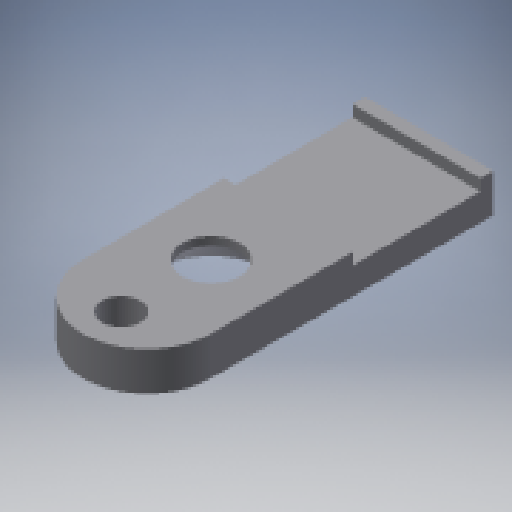
# Autodesk Inventor part: 24_0497_007
Saved by Autodesk Inventor 2024.3 (Build 283343000, 343)
## iProperties
Created: 2024-06-06
Part Number: 24_0497_007
Material: Allgemein
Document SubType Name: Modeling
Designer: Vogel
Density: 1 g/cm^3
Appearance: Vorgabe
Author: Vogel
Autodesk Inventor part; units mm, degrees
ref_plane "YZ Plane" through (0, 0, 0) normal (1, 0, 0) x (0, 1, 0)
ref_plane "XZ Plane" through (0, 0, 0) normal (0, 1, 0) x (-1, 0, 0)
ref_plane "XY Plane" through (0, 0, 0) normal (0, 0, 1) x (1, 0, 0)
sketch "Skizze1" plane through (0, 0, 0) normal (0, 0, 1) x (1, 0, 0)
  line L0 (-7, 0) -> (7, 0) projected
  line L1 (0, -30) -> (0, 5) projected
  line L2 (5, -20) -> (-5, -20)
  line L3 (-5, -20) -> (-5, 0)
  line L4 (-5, 0) -> (5, 0)
  line L5 (5, 0) -> (5, -20)
  line L6 (5, -20) -> (-5, 0) construction
  line L7 (-5, -20) -> (5, 0) construction
  arc A0 (-5, -20) -> (5, -20) centre (0, -20) ccw
  point P0 (0, 0)
  point P1 (0, -10)
  dimension "d0" = 10
  dimension "d1" = 20
  constraints: 12 end point, 2 midpoint, 2 parallel, 2 point on circle, 2 point on line, 2 tangent, 1 centre point, 1 horizontal, 1 perpendicular
  measures "d0" distance between parallel lines of L5 L3
  measures "d1" distance of L2.end L3.end
extrude "Extrusion1" add sketch "Skizze1" along normal blind 3
sketch "Skizze2" plane through (5, -20, 0) normal (1, 0, 0) x (0, 0, -1)
  line L0 (0, 0) -> (0, 20) projected
  line L1 (0, 20) -> (-3, 20) projected
  line L2 (-3, 0) -> (-3, 20) projected
  line L3 (0, 0) -> (-3, 0) projected
  line L4 (-3, 0) -> (-3, 20) projected
  line L5 (-3, 9.5) -> (-2.1, 9.5)
  line L6 (-2.1, 9.5) -> (-2.1, 19.5)
  line L7 (-2.1, 19.5) -> (-3, 19.5)
  line L8 (-3, 19.5) -> (-3, 9.5)
  point P0 (0, 20)
  point P1 (-2.55, 19.5)
  point P2 (-3, 19.5)
  dimension "d4" = 0.9
  dimension "d5" = 0.5
  dimension "d6" = 10
  constraints: 8 end point, 2 parallel, 1 horizontal, 1 midpoint, 1 perpendicular, 1 point on line
  measures "d4" distance of L5.start L5.end
  measures "d5" distance from line of point (-2.55, 19.5) L1
  measures "d6" distance of L5.end L6.end
extrude "Extrusion2" cut sketch "Skizze2" against normal through all contours L2 L7 L6 L5
sketch "Skizze4" plane through (0, 0, 0) normal (0, 0, -1) x (-1, 0, 0)
  arc A0 (-5, -20) -> (5, -20) centre (0, -20) ccw projected
  line L0 (5, 0) -> (5, -20) projected
  line L1 (-5, 0) -> (5, 0) projected
  line L2 (-5, -20) -> (-5, 0) projected
  line L3 (0, -32.4) -> (0, 5.4) projected
  line L4 (7, 0) -> (-7, 0) projected
  point P0 (0, 0)
  point P1 (0, -15)
  dimension "d9" = 5
  constraints: 1 coincident, 1 point on line
  measures "d9" distance of point (0, -15) point (0, -20)
hole "Bohrung1" at (0, -15, 0) direction (0, 0, 1) diameter 4.5 end through all countersink diameter 9.2 countersink angle 90
sketch "Skizze5" plane through (0, 0, 0) normal (0, 0, -1) x (-1, 0, 0)
  line L0 (0, -30) -> (0, 5) projected
  line L1 (7, 0) -> (-7, 0) projected
  circle A0 centre (0, -15) radius 4.6 projected
  point P0 (0, 0)
  point P1 (0, -22)
  dimension "d17" = 7
  constraints: 1 point on line
  measures "d17" distance of point (0, -22) A0.centre
hole "Bohrung2" at (0, -22, 0) direction (0, 0, 1) diameter 3 end through all
